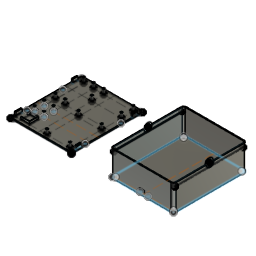
skylaser-base v9 (Autodesk Fusion 360 design; units mm, degrees)
Autodesk Fusion 360 part; units mm, degrees
sketch "Sketch1" plane through (0, 0, 0) normal (0, 0, 1) x (1, 0, 0)
  line L0 (-3, 0) -> (-117, 0)
  line L1 (-120, 3) -> (-120, 137)
  line L2 (-117, 140) -> (-3, 140)
  line L3 (0, 137) -> (0, 3)
  line L4 (-11, 0) -> (-11, 140) construction
  line L5 (-69, 0) -> (-69, 140) construction
  line L6 (-120, 132) -> (0, 132) construction
  line L7 (-120, 109) -> (0, 109) construction
  line L8 (-56.25, 0) -> (-56.25, 140) construction
  line L9 (-120, 8) -> (0, 8) construction
  line L10 (-120, 68) -> (0, 68) construction
  circle A0 centre (-56.25, 8) radius 2.5
  circle A1 centre (-56.25, 70) radius 2.5
  circle A2 centre (-11, 8) radius 2.5
  circle A3 centre (-11, 70) radius 2.5
  circle A4 centre (-11, 109) radius 2.5
  circle A5 centre (-11, 132) radius 2.5
  circle A6 centre (-11, 109) radius 1.25
  circle A7 centre (-11, 132) radius 1.25
  circle A8 centre (-56.25, 8) radius 1.25
  circle A9 centre (-56.25, 70) radius 1.25
  circle A10 centre (-11, 70) radius 1.25
  circle A11 centre (-11, 8) radius 1.25
  line L11 (-89, 0) -> (-89, 140) construction
  line L12 (-108.3, 0) -> (-108.3, 140) construction
  line L13 (-120, 76.5) -> (0, 76.5) construction
  circle A12 centre (-108.3, 132) radius 2.5
  circle A13 centre (-108.3, 76.5) radius 2.5
  circle A14 centre (-89, 76.5) radius 2.5
  circle A15 centre (-89, 132) radius 2.5
  circle A16 centre (-108.3, 76.5) radius 1.25
  circle A17 centre (-108.3, 132) radius 1.25
  circle A18 centre (-89, 76.5) radius 1.25
  circle A19 centre (-89, 132) radius 1.25
  line L14 (-120, 53.7388) -> (0, 53.7388) construction
  line L15 (-120, 35.2388) -> (0, 35.2388) construction
  line L16 (-107.5, 0) -> (-107.5, 140) construction
  circle A20 centre (-107.5, 53.7388) radius 2.5
  circle A21 centre (-107.5, 35.2388) radius 2.5
  circle A22 centre (-89, 35.2388) radius 2.5
  circle A23 centre (-89, 53.7388) radius 2.5
  circle A24 centre (-107.5, 35.2388) radius 1.25
  circle A25 centre (-107.5, 53.7388) radius 1.25
  circle A26 centre (-89, 35.2388) radius 1.25
  circle A27 centre (-89, 53.7388) radius 1.25
  line L17 (-90.5, 8) -> (-106, 8)
  line L18 (-106, 8) -> (-106, 24)
  line L19 (-106, 24) -> (-90.5, 24)
  line L20 (-90.5, 24) -> (-90.5, 8)
  line L21 (-89.5, 7) -> (-107, 7)
  line L22 (-107, 7) -> (-107, 25)
  line L23 (-107, 25) -> (-89.5, 25)
  line L24 (-89.5, 25) -> (-89.5, 7)
  arc A28 (-120, 3) -> (-117, 0) centre (-117, 3) ccw
  arc A29 (-117, 140) -> (-120, 137) centre (-117, 137) ccw
  arc A30 (0, 137) -> (-3, 140) centre (-3, 137) ccw
  arc A31 (-3, 0) -> (0, 3) centre (-3, 3) ccw
  line L25 (-3, 0) -> (-3, 140) construction
  line L26 (-117, 0) -> (-117, 140) construction
  circle A32 centre (-117, 99.934) radius 1.5
  circle A33 centre (-69, 132) radius 2.5
  circle A34 centre (-69, 109) radius 2.5
  circle A35 centre (-69, 132) radius 1.25
  circle A36 centre (-69, 109) radius 1.25
  line L27 (-120, 120) -> (-117, 120)
  line L28 (-117, 120) -> (-117, 129.7341)
  line L29 (-117, 129.7341) -> (-120, 129.7341)
  line L30 (-120, 129.7341) -> (-120, 120)
  line L31 (0, 120) -> (-3, 120)
  line L32 (-3, 120) -> (-3, 129.7341)
  line L33 (-3, 129.7341) -> (0, 129.7341)
  line L34 (0, 129.7341) -> (0, 120)
  line L35 (-120, 8) -> (-117, 8)
  line L36 (-117, 8) -> (-117, 20.1179)
  line L37 (-117, 20.1179) -> (-120, 20.1179)
  line L38 (-120, 20.1179) -> (-120, 8)
  line L39 (0, 10) -> (-3, 10)
  line L40 (-3, 10) -> (-3, 20.0425)
  line L41 (-3, 20.0425) -> (0, 20.0425)
  line L42 (0, 20.0425) -> (0, 10)
  circle A37 centre (-117, 29.5907) radius 1.5
  circle A38 centre (-3, 29.9611) radius 1.5
  circle A39 centre (-3, 99.9237) radius 1.5
  point P0 (-120, 0)
  point P1 (0, 140)
  dimension "d1" = 120
  dimension "d2" = 140
  dimension "d3" = 58
  dimension "d4" = 23
  dimension "d5" = 45.25
  dimension "d6" = 60
  dimension "d7" = 5
  dimension "d8" = 5
  dimension "d9" = 5
  dimension "d10" = 5
  dimension "d13" = 5
  dimension "d14" = 5
  dimension "d17" = 2.5
  dimension "d18" = 2.5
  dimension "d19" = 2.5
  dimension "d20" = 2.5
  dimension "d21" = 2.5
  dimension "d22" = 2.5
  dimension "d23" = 20
  dimension "d24" = 19.3
  dimension "d25" = 55.5
  dimension "d26" = 5
  dimension "d27" = 5
  dimension "d28" = 5
  dimension "d29" = 5
  dimension "d30" = 2.5
  dimension "d31" = 2.5
  dimension "d32" = 2.5
  dimension "d33" = 2.5
  dimension "d34" = 18.5
  dimension "d35" = 18.5
  dimension "d36" = 5
  dimension "d37" = 5
  dimension "d38" = 5
  dimension "d39" = 5
  dimension "d40" = 2.5
  dimension "d41" = 2.5
  dimension "d42" = 2.5
  dimension "d43" = 2.5
  dimension "d44" = 15.5
  dimension "d45" = 16
  dimension "d46" = -1
  dimension "d47" = 3
  dimension "d48" = 3
  dimension "d49" = 3
  dimension "d50" = 3
  dimension "d59" = 11
  dimension "d64" = 3
  dimension "d68" = 5
  dimension "d69" = 5
  dimension "d70" = 2.5
  dimension "d71" = 2.5
  dimension "d72" = 8
  dimension "d73" = 8
  dimension "d74" = 13
  dimension "d75" = 3
  dimension "d76" = 3
  dimension "d77" = 3
  constraint horizontal L0
  constraint vertical L1
  constraint horizontal L2
  constraint vertical L3
  constraint coincident L0 L4.start
  constraint coincident L2 L4.end
  constraint perpendicular L2 L4
  constraint coincident L0 L5.start
  constraint coincident L2 L5.end
  constraint perpendicular L2 L5
  constraint coincident L1 L6.start
  constraint coincident L3 L6.end
  constraint perpendicular L3 L6
  constraint coincident L1 L7.start
  constraint coincident L3 L7.end
  constraint perpendicular L3 L7
  constraint coincident L0 L8.start
  constraint coincident L2 L8.end
  constraint perpendicular L2 L8
  constraint coincident L1 L9.start
  constraint coincident L3 L9.end
  constraint perpendicular L3 L9
  constraint coincident L1 L10.start
  constraint coincident L3 L10.end
  constraint perpendicular L3 L10
  constraint coincident L8 A0.centre
  constraint coincident L9 A0.centre
  constraint midpoint L8 A1.centre
  constraint coincident L4 A2.centre
  constraint coincident L9 A2.centre
  constraint midpoint L4 A3.centre
  constraint coincident L4 A4.centre
  constraint coincident L7 A4.centre
  constraint coincident L6 A5.centre
  constraint coincident L4 A5.centre
  constraint concentric A4 A6
  constraint concentric A5 A7
  constraint concentric A0 A8
  constraint concentric A1 A9
  constraint concentric A3 A10
  constraint concentric A2 A11
  constraint coincident L0 L11.start
  constraint coincident L2 L11.end
  constraint perpendicular L2 L11
  constraint coincident L0 L12.start
  constraint coincident L2 L12.end
  constraint perpendicular L2 L12
  constraint coincident L1 L13.start
  constraint coincident L3 L13.end
  constraint perpendicular L3 L13
  constraint coincident L6 A12.centre
  constraint coincident L12 A12.centre
  constraint coincident L12 A13.centre
  constraint coincident L13 A13.centre
  constraint coincident L11 A14.centre
  constraint coincident L13 A14.centre
  constraint coincident L6 A15.centre
  constraint coincident L11 A15.centre
  constraint concentric A13 A16
  constraint concentric A12 A17
  constraint concentric A14 A18
  constraint concentric A15 A19
  constraint coincident L1 L14.start
  constraint coincident L3 L14.end
  constraint perpendicular L3 L14
  constraint coincident L1 L15.start
  constraint coincident L3 L15.end
  constraint perpendicular L3 L15
  constraint coincident L0 L16.start
  constraint coincident L2 L16.end
  constraint perpendicular L2 L16
  constraint coincident L14 A20.centre
  constraint coincident L16 A20.centre
  constraint coincident L15 A21.centre
  constraint coincident L16 A21.centre
  constraint coincident L15 A22.centre
  constraint coincident L11 A22.centre
  constraint coincident L14 A23.centre
  constraint coincident L11 A23.centre
  constraint concentric A21 A24
  constraint concentric A20 A25
  constraint concentric A22 A26
  constraint concentric A23 A27
  constraint horizontal L17
  constraint vertical L18
  constraint horizontal L19
  constraint vertical L20
  constraint coincident L9 L17.start
  constraint coincident P0 L0
  constraint coincident P0 L1
  constraint tangent L0 A28
  constraint tangent L1 A28
  constraint tangent L2 A29
  constraint tangent L1 A29
  constraint coincident P1 L2
  constraint coincident P1 L3
  constraint tangent L2 A30
  constraint tangent L3 A30
  constraint coincident origin L3
  constraint coincident origin L0
  constraint tangent L3 A31
  constraint tangent L0 A31
  constraint coincident L26 A32.centre
  constraint coincident L6 A33.centre
  constraint coincident L5 A33.centre
  constraint coincident L7 A34.centre
  constraint coincident L5 A34.centre
  constraint concentric A33 A35
  constraint concentric A34 A36
  constraint horizontal L27
  constraint vertical L28
  constraint horizontal L29
  constraint vertical L30
  constraint coincident L26 L28.end
  constraint coincident L1 L27.start
  constraint horizontal L31
  constraint vertical L32
  constraint horizontal L33
  constraint vertical L34
  constraint coincident L25 L32.end
  constraint coincident L3 L31.start
  constraint horizontal L35
  constraint vertical L36
  constraint horizontal L37
  constraint vertical L38
  constraint coincident L26 L36.end
  constraint horizontal L39
  constraint vertical L40
  constraint horizontal L41
  constraint vertical L42
  constraint coincident L3 L39.start
  constraint coincident L26 A37.centre
  constraint coincident L25 A38.centre
  constraint coincident L25 A39.centre
  measures "d1" distance of origin P0
  measures "d2" distance of origin P1
  measures "d3" distance of L4 L5
  measures "d4" distance of L6 L7
  measures "d5" distance of L4 L8
  measures "d6" distance of L9 L10
  measures "d7" diameter of A0
  measures "d8" diameter of A1
  measures "d9" diameter of A2
  measures "d10" diameter of A3
  measures "d13" diameter of A4
  measures "d14" diameter of A5
  measures "d17" diameter of A6
  measures "d18" diameter of A7
  measures "d19" diameter of A8
  measures "d20" diameter of A9
  measures "d21" diameter of A10
  measures "d22" diameter of A11
  measures "d23" distance of L5 L11
  measures "d24" distance of L11 L12
  measures "d25" distance of L6 L13
  measures "d26" diameter of A12
  measures "d27" diameter of A13
  measures "d28" diameter of A14
  measures "d29" diameter of A15
  measures "d30" diameter of A16
  measures "d31" diameter of A17
  measures "d32" diameter of A18
  measures "d33" diameter of A19
  measures "d34" distance of L14 L15
  measures "d35" distance of L11 L16
  measures "d36" diameter of A20
  measures "d37" diameter of A21
  measures "d38" diameter of A22
  measures "d39" diameter of A23
  measures "d40" diameter of A24
  measures "d41" diameter of A25
  measures "d42" diameter of A26
  measures "d43" diameter of A27
  measures "d44" distance of L17.start L17.end
  measures "d45" distance of L17.start L19.end
  measures "d47" radius of A28
  measures "d48" radius of A29
  measures "d49" radius of A30
  measures "d50" radius of A31
  measures "d59" distance of L3 L4
  measures "d64" diameter of A32
  measures "d68" diameter of A33
  measures "d69" diameter of A34
  measures "d70" diameter of A35
  measures "d71" diameter of A36
  measures "d72" distance of L2 L6
  measures "d73" distance of L0 L9
  measures "d74" distance of L1 L22
  measures "d75" diameter of A37
  measures "d76" diameter of A38
  measures "d77" diameter of A39
extrude "Extrude1" add sketch "Sketch1" along normal blind 2 contours L0 L1 L2 L3 A28 A29 A30 A31 L27 L28 L29 L31 L32 L33 L35 L36 L37 L39 L40 L41 | L3 L39 L40 L41 L42 | L1 L35 L36 L37 L38 | L3 L31 L32 L33 L34 | L1 L27 L28 L29 L30 | A0 | A1 | A2 | A3 | A4 | A5 | A6 | A7 | A8 | A9 | A10 | A11 | A12 | A13 | A14 | A15 | A16 | A17 | A18 | A19 | A20 | A21 | A22 | A23 | A24 | A25 | A26 | A27 | L17 L18 L19 L20 | L21 L22 L23 L24 | A32 | A33 | A34 | A35 | A36 | A37 | A38 | A39 makes body 1
extrude "Extrude2" add sketch "Sketch1" along normal blind 10 contours A0 | A1 | A2 | A3 | A4 | A5 | A12 | A13 | A14 | A15 | A20 | A21 | A22 | A23 | A33 | A34 bodies 1
extrude "Extrude3" add sketch "Sketch1" along normal blind 6 contours L21 L22 L23 L24 bodies 1
sketch "Sketch2" plane through (-107, 0, 0) normal (-1, 0, 0) x (0, -1, 0)
  line L0 (-25, 2) -> (-7, 2)
  line L1 (-7, 2) -> (-7, 6)
  line L2 (-7, 6) -> (-25, 6)
  line L3 (-25, 6) -> (-25, 2)
  line L4 (-20.0162, 6) -> (-8.0568, 6)
  line L5 (-8.0568, 6) -> (-8.0568, 2)
  line L6 (-8.0568, 2) -> (-20.0162, 2)
  line L7 (-20.0162, 2) -> (-20.0162, 6)
  constraint horizontal L4
  constraint vertical L5
  constraint horizontal L6
  constraint vertical L7
  constraint coincident L0 L5.end
  constraint coincident L2 L4.start
extrude "Extrude4" cut sketch "Sketch2" against normal blind 4 contours L0 L2 L4 L5 L6 L7 bodies 1
extrude "Extrude5" cut sketch "Sketch1" along normal blind 10 contours A32 | A37 | A38 | A39 bodies 1
extrude "Extrude6" add sketch "Sketch1" along normal blind 8 contours L3 L39 L40 L41 L42 | L1 L35 L36 L37 L38 | L3 L31 L32 L33 L34 | L1 L27 L28 L29 L30 bodies 1
sketch "Sketch3" plane through (0, 0, 0) normal (1, 0, 0) x (0, 1, 0)
  line L0 (3, 0) -> (137, 0)
  line L1 (137, 0) -> (137, 2)
  line L2 (137, 2) -> (129.7341, 2)
  line L3 (129.7341, 2) -> (129.7341, 8)
  line L4 (129.7341, 8) -> (120, 8)
  line L5 (120, 8) -> (120, 2)
  line L6 (120, 2) -> (20.0425, 2)
  line L7 (20.0425, 2) -> (20.0425, 8)
  line L8 (20.0425, 8) -> (10, 8)
  line L9 (10, 8) -> (10, 2)
  line L10 (10, 2) -> (3, 2)
  line L11 (3, 2) -> (3, 0)
  line L12 (10, 8) -> (20.0425, 8)
  line L13 (20.0425, 8) -> (20.0425, 7)
  line L14 (20.0425, 7) -> (10, 7)
  line L15 (10, 7) -> (10, 8)
  line L16 (120, 8) -> (129.7341, 8)
  line L17 (129.7341, 8) -> (129.7341, 7)
  line L18 (129.7341, 7) -> (120, 7)
  line L19 (120, 7) -> (120, 8)
  dimension "d80" = 1
  dimension "d81" = 1
  constraint horizontal L12
  constraint vertical L13
  constraint horizontal L14
  constraint vertical L15
  constraint coincident L8.end L9.start
  constraint horizontal L16
  constraint vertical L17
  constraint horizontal L18
  constraint vertical L19
  constraint coincident L4.end L5.start
  measures "d80" distance of L8.end L14.end
  measures "d81" distance of L4.end L18.end
extrude "Extrude7" add sketch "Sketch3" along normal blind 0.5 contours L7 L8 L9 L12 L13 L14 L15 | L3 L4 L5 L16 L17 L18 L19 bodies 1
fillet "Fillet1" radius 1 1 edges at (0.5, 124.8671, 8) on bodies 1
fillet "Fillet2" radius 1 1 edges at (0.5, 15.0213, 8) on bodies 1
sketch "Sketch4" plane through (-120, 0, 0) normal (-1, 0, 0) x (0, -1, 0)
  line L0 (-137, 0) -> (-3, 0)
  line L1 (-3, 0) -> (-3, 2)
  line L2 (-3, 2) -> (-8, 2)
  line L3 (-8, 2) -> (-8, 8)
  line L4 (-8, 8) -> (-20.1179, 8)
  line L5 (-20.1179, 8) -> (-20.1179, 2)
  line L6 (-20.1179, 2) -> (-120, 2)
  line L7 (-120, 2) -> (-120, 8)
  line L8 (-120, 8) -> (-129.7341, 8)
  line L9 (-129.7341, 8) -> (-129.7341, 2)
  line L10 (-129.7341, 2) -> (-137, 2)
  line L11 (-137, 2) -> (-137, 0)
  line L12 (-129.7341, 8) -> (-120, 8)
  line L13 (-120, 8) -> (-120, 7)
  line L14 (-120, 7) -> (-129.7341, 7)
  line L15 (-129.7341, 7) -> (-129.7341, 8)
  line L16 (-20.1179, 8) -> (-8, 8)
  line L17 (-8, 8) -> (-8, 7)
  line L18 (-8, 7) -> (-20.1179, 7)
  line L19 (-20.1179, 7) -> (-20.1179, 8)
  dimension "d88" = 1
  dimension "d89" = 1
  constraint horizontal L12
  constraint vertical L13
  constraint horizontal L14
  constraint vertical L15
  constraint coincident L8.end L9.start
  constraint horizontal L16
  constraint vertical L17
  constraint horizontal L18
  constraint vertical L19
  constraint coincident L4.end L5.start
  measures "d88" distance of L8.end L14.end
  measures "d89" distance of L4.end L18.end
extrude "Extrude8" add sketch "Sketch4" along normal blind 0.5 contours L7 L8 L9 L12 L13 L14 L15 | L3 L4 L5 L16 L17 L18 L19 bodies 1
fillet "Fillet3" radius 1 1 edges at (-120.5, 14.059, 8) on bodies 1
fillet "Fillet4" radius 1 1 edges at (-120.5, 124.8671, 8) on bodies 1
sketch "Sketch5" plane through (0, 0, 0) normal (0, 0, 1) x (1, 0, 0)
sketch "Sketch6" plane through (0, 0, 0) normal (0, 0, 1) x (1, 0, 0)
  line L0 (83, 0) -> (197, 0)
  line L1 (200, 3) -> (200, 137)
  line L2 (197, 140) -> (83, 140)
  line L3 (80, 137) -> (80, 3)
  arc A0 (200, 137) -> (197, 140) centre (197, 137) ccw
  arc A1 (197, 0) -> (200, 3) centre (197, 3) ccw
  arc A2 (83, 140) -> (80, 137) centre (83, 137) ccw
  arc A3 (80, 3) -> (83, 0) centre (83, 3) ccw
  line L4 (78, 137) -> (78, 3)
  arc A4 (78, 3) -> (83, -2) centre (83, 3) ccw
  line L5 (83, -2) -> (197, -2)
  arc A5 (197, -2) -> (202, 3) centre (197, 3) ccw
  line L6 (202, 3) -> (202, 137)
  arc A6 (202, 137) -> (197, 142) centre (197, 137) ccw
  line L7 (197, 142) -> (83, 142)
  arc A7 (83, 142) -> (78, 137) centre (83, 137) ccw
  line L8 (140, 140) -> (140, 0) construction
  line L9 (80, 2.4) -> (200, 2.4) construction
  circle A8 centre (132.25, 2.4) radius 2.5
  circle A9 centre (147.75, 2.4) radius 2.5
  circle A10 centre (132.25, 2.4) radius 1.25
  circle A11 centre (147.75, 2.4) radius 1.25
  point P0 (80, 0)
  point P1 (200, 0)
  point P2 (80, 140)
  dimension "d96" = 120
  dimension "d97" = 140
  dimension "d98" = 3
  dimension "d99" = 3
  dimension "d100" = 3
  dimension "d101" = 3
  dimension "d102" = 2
  dimension "d121" = 5
  dimension "d122" = 5
  dimension "d123" = 7.75
  dimension "d124" = 7.75
  dimension "d125" = 2.4
  dimension "d126" = 2.5
  dimension "d127" = 2.5
  constraint horizontal L0
  constraint vertical L1
  constraint horizontal L2
  constraint vertical L3
  constraint tangent L1 A0
  constraint tangent L2 A0
  constraint coincident P1 L0
  constraint coincident P1 L1
  constraint tangent L0 A1
  constraint tangent L1 A1
  constraint coincident P2 L2
  constraint coincident P2 L3
  constraint tangent L2 A2
  constraint tangent L3 A2
  constraint coincident P0 L0
  constraint coincident P0 L3
  constraint tangent L0 A3
  constraint tangent L3 A3
  constraint midpoint L2 L8.start
  constraint midpoint L0 L8.end
  constraint coincident L3 L9.start
  constraint coincident L1 L9.end
  constraint perpendicular L1 L9
  constraint coincident L9 A8.centre
  constraint coincident L9 A9.centre
  constraint concentric A8 A10
  constraint concentric A9 A11
  measures "d96" distance of P0 P1
  measures "d97" distance of P0 P2
  measures "d98" radius of A0
  measures "d99" radius of A1
  measures "d100" radius of A2
  measures "d101" radius of A3
  measures "d121" diameter of A8
  measures "d122" diameter of A9
  measures "d123" distance of L8 A9.centre
  measures "d124" distance of L8 A8.centre
  measures "d125" distance of L0 L9
  measures "d126" diameter of A10
  measures "d127" diameter of A11
extrude "Extrude9" add sketch "Sketch6" along normal blind 1 separate body contours L0 L1 L2 L3 A0 A1 A2 A3 A8 A9 | L0 A8 | L0 A8 | L0 A9 | L0 A9 | L4 A4 L5 A5 L6 A6 L7 A7 | A10 | A11 makes body 2
extrude "Extrude10" add sketch "Sketch6" along normal blind 50 contours L0 A8 | L0 A9 | L4 A4 L5 A5 L6 A6 L7 A7 picked at (132.3679, -0.025) picked at (147.8679, -0.025) bodies 2
sketch "Sketch7" plane through (200, 0, 0) normal (-1, 0, 0) x (0, -1, 0)
  line L0 (-137, 1) -> (-3, 1)
  line L1 (-3, 1) -> (-3, 50)
  line L2 (-3, 50) -> (-137, 50)
  line L3 (-137, 50) -> (-137, 1)
  line L4 (-137, 42) -> (-3, 42) construction
  line L5 (-137, 42) -> (-3, 42)
  line L6 (-3, 42) -> (-3, 43.5)
  line L7 (-3, 43.5) -> (-137, 43.5)
  line L8 (-137, 43.5) -> (-137, 42)
  circle A0 centre (-70, 50) radius 7.5
  dimension "d107" = 8
  dimension "d108" = 1.5
  dimension "d115" = 15
  constraint coincident L3 L4.start
  constraint coincident L1 L4.end
  constraint perpendicular L1 L4
  constraint horizontal L5
  constraint vertical L6
  constraint horizontal L7
  constraint vertical L8
  constraint coincident L1 L6.end
  constraint midpoint L2 A0.centre
  measures "d107" distance of L2 L4
  measures "d108" distance of L5 L7
  measures "d115" diameter of A0
extrude "Extrude11" cut sketch "Sketch7" against normal blind 0.5 contours L1 L3 L5 L6 L7 L8 A0 | L7 A0 bodies 2
sketch "Sketch8" plane through (80, 0, 0) normal (1, 0, 0) x (0, 1, 0)
  line L0 (3, 1) -> (137, 1)
  line L1 (137, 1) -> (137, 50)
  line L2 (137, 50) -> (3, 50)
  line L3 (3, 50) -> (3, 1)
  line L4 (3, 42) -> (137, 42)
  line L5 (137, 42) -> (137, 43.5)
  line L6 (137, 43.5) -> (3, 43.5)
  line L7 (3, 43.5) -> (3, 42)
  circle A0 centre (70, 50) radius 7.5
  dimension "d111" = 8
  dimension "d112" = 1.5
  dimension "d118" = 15
  constraint horizontal L4
  constraint vertical L5
  constraint horizontal L6
  constraint vertical L7
  constraint coincident L1 L5.end
  constraint coincident L3 L4.start
  constraint midpoint L2 A0.centre
  measures "d111" distance of L2 L4
  measures "d112" distance of L4 L6
  measures "d118" diameter of A0
extrude "Extrude12" cut sketch "Sketch8" against normal blind 0.5 contours L1 L3 L4 L5 L6 L7 A0 | L6 A0 bodies 2
extrude "Extrude13" cut sketch "Sketch7" against normal blind 5 contours L2 L7 A0 | L7 A0 bodies 2
extrude "Extrude14" cut sketch "Sketch8" against normal blind 5 contours L2 L6 A0 | L6 A0 bodies 2
extrude "Extrude15" add sketch "Sketch6" along normal blind 6 contours L0 A8 | L0 A9 picked at (132.2811, 0.3845) picked at (147.7811, 0.3845) bodies 2
sketch "Sketch9" plane through (0, -2, 0) normal (0, -1, 0) x (1, 0, 0)
  line L0 (83, 0) -> (197, 0)
  line L1 (197, 0) -> (197, 50)
  line L2 (197, 50) -> (83, 50)
  line L3 (83, 50) -> (83, 0)
  line L4 (140, 50) -> (140, 0) construction
  line L5 (145, 6.4) -> (135, 6.4)
  line L6 (135, 6.4) -> (135, 10.4)
  line L7 (135, 10.4) -> (145, 10.4)
  line L8 (145, 10.4) -> (145, 6.4)
  line L9 (145, 6.4) -> (135, 10.4) construction
  line L10 (135, 6.4) -> (145, 10.4) construction
  line L11 (83, 0) -> (197, 0)
  point P0 (140, 8.4)
  dimension "d130" = 10
  dimension "d131" = 4
  dimension "d132" = 6.4
  constraint midpoint L2 L4.start
  constraint midpoint L0 L4.end
  constraint horizontal L5
  constraint perpendicular L5 L6
  constraint parallel L5 L7
  constraint parallel L6 L8
  constraint coincident L9 P0
  constraint coincident L10 P0
  constraint coincident L4 P0
  measures "d130" distance of L6.end L7.end
  measures "d131" distance of L5.end L6.end
  measures "d132" distance of L5 L11
extrude "Extrude16" cut sketch "Sketch9" against normal blind 15 contours L5 L6 L7 L8 bodies 2
equation "d123 = ( 15.5 / 2 ) * 1 mm"
equation "d124 = ( 15.5 / 2 ) * 1 mm"
equation "d132 = 5 mm + 1.4 mm"
